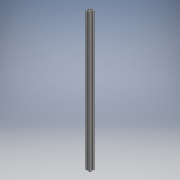
# Autodesk Inventor part: maker-beam-300x10x10mm
Saved by Autodesk Inventor 2016 (Build 200138000, 138)
## iProperties
Created: 2015-10-07
Part Number: maker-beam-300x10x10mm
Material: Generic
Document SubType Name: Modeling
Designer: Thomas
Density: 1 g/cm^3
Appearance: Default
Author: Thomas
Autodesk Inventor part; units mm, degrees
ref_plane "YZ Plane" through (0, 0, 0) normal (1, 0, 0) x (0, 1, 0)
ref_plane "XZ Plane" through (0, 0, 0) normal (0, 1, 0) x (-1, 0, 0)
ref_plane "XY Plane" through (0, 0, 0) normal (0, 0, 1) x (1, 0, 0)
sketch "Sketch1" plane through (0, 0, 0) normal (0, 0, 1) x (1, 0, 0)
  line L0 (-4.4697, -5.5303) -> (4.4697, 5.5303) construction
  line L1 (5.5303, 4.4697) -> (-5, -4.0411) construction
  line L2 (4.4697, -5.5303) -> (-4.4697, 5.5303) construction
  line L3 (-5.5303, 4.4697) -> (5.5303, -4.4697) construction
  line L4 (-5, -5) -> (-5, -3.9393)
  line L5 (-5, 3.9393) -> (-5, 5)
  line L6 (5, 5) -> (5, 3.9393)
  line L7 (5, -3.9393) -> (5, -5)
  line L8 (-5, 5) -> (-3.9393, 5)
  line L9 (3.9393, 5) -> (5, 5)
  line L10 (5, -5) -> (3.9393, -5)
  line L11 (-3.9393, -5) -> (-5, -5)
  line L12 (-2.6893, 3.75) -> (-0.4393, 1.5)
  line L13 (2.6893, 3.75) -> (0.4393, 1.5)
  line L14 (-1.5, -0.4393) -> (-3.75, -2.6893)
  line L15 (-1.5, 0.4393) -> (-3.75, 2.6893)
  line L16 (2.6893, -3.75) -> (0.4393, -1.5)
  line L17 (-2.6893, -3.75) -> (-0.4393, -1.5)
  line L18 (1.5, 0.4393) -> (3.75, 2.6893)
  line L19 (1.5, -0.4393) -> (3.75, -2.6893)
  line L20 (5, -5) -> (-5, 5) construction
  line L21 (-5, -5) -> (5, 5) construction
  line L22 (3.75, -3.75) -> (-3.75, 3.75) construction
  line L23 (-3.75, -3.75) -> (3.75, 3.75) construction
  line L24 (1.5, -5) -> (-1.5, 5) construction
  line L25 (-1.5, -5) -> (1.5, 5) construction
  line L26 (5, -1.5) -> (-5, 1.5) construction
  line L27 (-5, -1.5) -> (5, 1.5) construction
  line L28 (-5, 1.5) -> (-3.75, 1.5)
  line L29 (-3.75, -1.5) -> (-5, -1.5)
  line L30 (-3.75, -2.6893) -> (-3.75, -1.5)
  line L31 (-3.75, 1.5) -> (-3.75, 2.6893)
  line L32 (-5, -5) -> (-5, -1.5)
  line L33 (-5, 1.5) -> (-5, 5)
  line L34 (-5, 5) -> (-1.5, 5)
  line L35 (1.5, 5) -> (5, 5)
  line L36 (-1.5, 3.75) -> (-1.5, 5)
  line L37 (-2.6893, 3.75) -> (-1.5, 3.75)
  line L38 (1.5, 3.75) -> (2.6893, 3.75)
  line L39 (1.5, 5) -> (1.5, 3.75)
  line L40 (3.75, 1.5) -> (5, 1.5)
  line L41 (3.75, 2.6893) -> (3.75, 1.5)
  line L42 (3.75, -1.5) -> (3.75, -2.6893)
  line L43 (5, 5) -> (5, 1.5)
  line L44 (5, -1.5) -> (5, -5)
  line L45 (5, -1.5) -> (3.75, -1.5)
  line L46 (-0.45, 1.5) -> (0.45, 1.5)
  line L47 (-1.5, -5) -> (-1.5, -3.75)
  line L48 (-1.5, -0.45) -> (-1.5, 0.45)
  line L49 (1.5, 0.45) -> (1.5, -0.45)
  line L50 (2.6893, -3.75) -> (1.5, -3.75)
  line L51 (5, -5) -> (1.5, -5)
  line L52 (-1.5, -5) -> (-5, -5)
  line L53 (1.5, -3.75) -> (1.5, -5)
  line L54 (0.45, -1.5) -> (-0.45, -1.5)
  line L55 (-1.5, -3.75) -> (-2.6893, -3.75)
  point P0 (0, 0)
  point P1 (0, 0)
  dimension "d0" = 10
  dimension "d7" = 1.5
  dimension "d8" = 1.5
  dimension "d9" = 7.5
  dimension "d10" = 7.5
  dimension "d11" = 10
  dimension "d12" = 3
  dimension "d13" = 3
  constraints: 112 end point, 50 parallel, 18 point on line, 12 midpoint, 12 perpendicular, 9 horizontal
  measures "d0" distance of L7.end L6.start
  measures "d7" distance of L0.end L1.start
  measures "d8" distance of L3.start L2.end
  measures "d9" distance of L22.end L23.end
  measures "d10" distance of L23.end L22.start
  measures "d11" distance of L5.end L21.end
  measures "d12" distance of L24.end L25.end
  measures "d13" distance of L27.start L26.end
extrude "Extrusion1" add sketch "Sketch1" along normal blind 300
equation "\"d8\" = d7"
equation "\"d10\" = d9"
equation "\"d11\" = d0"
equation "\"d4\" = 0.5 * d0"
equation "\"d5\" = 0.5 * d0"
equation "\"d6\" = 0.5 * d0"
body "Solid1"
